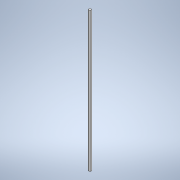
# Autodesk Inventor part: SP17V1 Varilla Pedal
Saved by Autodesk Inventor 2021.2 (Build 252289000, 289)
## iProperties
Created: 2026-06-16
Part Number: SP17V1 Varilla Pedal
Material: Generic
Document SubType Name: Modeling
Designer: nelso
Density: 1 g/cm^3
Appearance: Default
Author: nelso
Autodesk Inventor part; units mm, degrees
ref_plane "YZ Plane" through (0, 0, 0) normal (1, 0, 0) x (0, 1, 0)
ref_plane "XZ Plane" through (0, 0, 0) normal (0, 1, 0) x (-1, 0, 0)
ref_plane "XY Plane" through (0, 0, 0) normal (0, 0, 1) x (1, 0, 0)
sketch "Sketch1" plane through (0, 0, 0) normal (0, 1, 0) x (-1, 0, 0)
  circle A0 centre (0, 0) radius 6.35
  line L0 (0, -9.2376) -> (-8, -4.6188)
  line L1 (-8, -4.6188) -> (-8, 4.6188)
  line L2 (-8, 4.6188) -> (0, 9.2376)
  line L3 (0, 9.2376) -> (8, 4.6188)
  line L4 (8, 4.6188) -> (8, -4.6188)
  line L5 (8, -4.6188) -> (0, -9.2376)
  dimension "d0" = 12.7
  dimension "d3" = 16
  constraints: 12 end point, 2 coincident, 1 centre point, 13 other
  measures "d0" diameter of A0
  measures "d3" distance between parallel lines of L1 L4
extrude "Extrusion1" add sketch "Sketch1" along normal mid plane 1050 contours A0 | L0 L1 L2 L3 L4 L5
body "Solid1"
